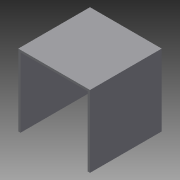
# Autodesk Inventor part: AutoBucket
Saved by Autodesk Inventor 2013 (Build 170138000, 138)
## iProperties
Created: 2014-02-01
Part Number: AutoBucket
Material: Generic
Document SubType Name: Modeling
Designer: nojessen
Density: 1 g/cm^3
Author: nojessen
Autodesk Inventor part; units mm, degrees
ref_plane "YZ Plane" through (0, 0, 0) normal (1, 0, 0) x (0, 1, 0)
ref_plane "XZ Plane" through (0, 0, 0) normal (0, 1, 0) x (-1, 0, 0)
ref_plane "XY Plane" through (0, 0, 0) normal (0, 0, 1) x (1, 0, 0)
sketch "Sketch1" plane through (0, 0, 0) normal (0, 0, 1) x (1, 0, 0)
  line L0 (0, 0) -> (50.8, 0)
  line L1 (50.8, 0) -> (50.8, 50.8)
  line L2 (50.8, 50.8) -> (0, 50.8)
  line L3 (0, 50.8) -> (0, 0)
  dimension "d0" = 50.8
  dimension "d2" = 50.8
  constraints: 8 end point, 2 parallel, 1 horizontal, 1 perpendicular
  measures "d0" distance of L1.end L2.end
  measures "d2" distance of L0.end L1.end
extrude "Extrusion1" add sketch "Sketch1" along normal blind 1.5875
sketch "Sketch2" plane through (0, 0, 1.5875) normal (0, 0, 1) x (1, 0, 0)
  line L0 (0, 0) -> (50.8, 0) projected
  line L1 (0, 50.8) -> (1.5875, 50.8)
  line L2 (1.5875, 49.2125) -> (1.5875, 0)
  line L3 (1.5875, 0) -> (0, 0)
  line L4 (0, 0) -> (0, 50.8)
  line L5 (0, 50.8) -> (50.8, 50.8)
  line L6 (50.8, 50.8) -> (50.8, 49.2125)
  line L7 (49.2125, 49.2125) -> (1.5875, 49.2125)
  line L8 (0, 49.2125) -> (0, 50.8)
  line L9 (50.8, 50.8) -> (49.2125, 50.8)
  line L10 (49.2125, 49.2125) -> (49.2125, 0)
  line L11 (49.2125, 0) -> (50.8, 0)
  line L12 (50.8, 0) -> (50.8, 50.8)
  dimension "d5" = 1.5875
  dimension "d6" = 50.8
  dimension "d7" = 1.5875
  dimension "d8" = 1.5875
  constraints: 24 end point, 6 parallel, 3 horizontal, 3 perpendicular, 2 point on line
  measures "d5" distance of L2.end L3.end
  measures "d6" distance of L6.end L8.start
  measures "d7" distance between parallel lines of L7 L5
  measures "d8" distance of L11.end L10.end
extrude "Extrusion2" add sketch "Sketch2" along normal blind 49.2125 contours L4 L1 L5 L6 L12 L0 L10 L7 L2
body "Solid1"
